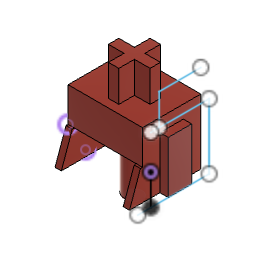
stem v4 (Autodesk Fusion 360 design; units mm, degrees)
Autodesk Fusion 360 part; units mm, degrees
note: some values were not read from the file. Set by a fixed rule: which sketch regions a step uses.
sketch "Sketch1" plane through (0, 0, 0) normal (0, 1, 0) x (1, 0, 0)
  line L0 (0, 0) -> (7.15, 0)
  line L1 (7.15, 0) -> (7.15, -3.3)
  line L2 (7.15, -3.3) -> (0, -3.3)
  line L3 (0, -3.3) -> (0, 0)
  line L4 (0, 0) -> (0.6, 0)
  line L5 (0.6, 0) -> (0.6, 2.95)
  line L6 (0.6, 2.95) -> (0, 2.95)
  line L7 (0, 2.95) -> (0, 0)
  line L8 (7.15, 0) -> (6.55, 0)
  line L9 (6.55, 0) -> (6.55, 2.95)
  line L10 (6.55, 2.95) -> (7.15, 2.95)
  line L11 (7.15, 2.95) -> (7.15, 0)
  dimension "d1" = 7.15
  dimension "d2" = 3.3
  dimension "d3" = 0.6
  dimension "d4" = 2.95
  dimension "d5" = 0.6
  dimension "d6" = 2.95
  constraint horizontal L0
  constraint vertical L1
  constraint horizontal L2
  constraint vertical L3
  constraint coincident L0.start L3.end
  constraint horizontal L4
  constraint vertical L5
  constraint horizontal L6
  constraint vertical L7
  constraint horizontal L8
  constraint vertical L9
  constraint horizontal L10
  constraint vertical L11
  measures "d1" distance of L0.start L0.end
  measures "d2" distance of L0.start L2.end
  measures "d3" distance of L0.start L4.end
  measures "d4" distance of L0.start L6.end
  measures "d5" distance of L0.end L8.end
  measures "d6" distance of L0.end L10.end
extrude "Extrude1" add sketch "Sketch1" along normal blind 5.6
sketch "Sketch2" plane through (7.15, 0, 0) normal (1, 0, 0) x (0, 1, 0)
  line L0 (0, 3.3) -> (0, -2.95)
  line L1 (0, -2.95) -> (5.6, -2.95)
  line L2 (5.6, -2.95) -> (5.6, 3.3)
  line L3 (5.6, 3.3) -> (0, 3.3)
  line L4 (1.675, -2.95) -> (3.925, -2.95)
  line L5 (3.925, -2.95) -> (3.925, 2.05)
  line L6 (3.925, 2.05) -> (1.675, 2.05)
  line L7 (1.675, 2.05) -> (1.675, -2.95)
  point P0 (2.8, 0)
  dimension "d12" = 2.25
  dimension "d13" = 5
  constraint horizontal L4
  constraint vertical L5
  constraint horizontal L6
  constraint vertical L7
  constraint coincident L1 L4.start
  measures "d12" distance of L4.start L4.end
  measures "d13" distance of L4.start L6.end
extrude "Extrude2" add sketch "Sketch2" along normal blind 0.8 contours L1 L4 L5 L6 L7
sketch "Sketch3" plane through (0, 0, 0) normal (-1, 0, 0) x (0, -1, 0)
  line L0 (0, -2.95) -> (0, 3.3)
  line L1 (0, 3.3) -> (-5.6, 3.3)
  line L2 (-5.6, 3.3) -> (-5.6, -2.95)
  line L3 (-5.6, -2.95) -> (0, -2.95)
  line L4 (-1.675, -2.5004) -> (-1.675, -2.95)
  line L5 (-1.675, -2.95) -> (-3.925, -2.95)
  line L6 (-3.925, -2.95) -> (-3.925, -2.5004)
  line L7 (-1.675, -2.95) -> (-3.925, -2.95)
  line L8 (-3.925, -2.95) -> (-3.925, 2.05)
  line L9 (-3.925, 2.05) -> (-1.675, 2.05)
  line L10 (-1.675, 2.05) -> (-1.675, -2.95)
  point P0 (-2.8, -0.0004)
  dimension "d19" = 2.25
  dimension "d20" = 5
  constraint vertical L4
  constraint horizontal L5
  constraint vertical L6
  constraint horizontal L7
  constraint vertical L8
  constraint horizontal L9
  constraint vertical L10
  measures "d19" distance of L6.end L4.start
  measures "d20" distance of L4.end L9.end
extrude "Extrude3" add sketch "Sketch3" along normal blind 0.8 contours L3 L4 L5 L6 L7 L8 L9 L10
sketch "Sketch4" plane through (0, 0, 0) normal (0, -1, 0) x (1, 0, 0)
  line L0 (0.6, -2.95) -> (0.6, 0)
  line L1 (0.6, 0) -> (6.55, 0)
  line L2 (6.55, 0) -> (6.55, -2.95)
  line L3 (6.55, -2.95) -> (7.15, -2.95)
  line L4 (7.15, -2.95) -> (7.15, 3.3)
  line L5 (7.15, 3.3) -> (0, 3.3)
  line L6 (0, 3.3) -> (0, -2.95)
  line L7 (0, -2.95) -> (0.6, -2.95)
  line L8 (0, 0) -> (0.6, 0)
  line L9 (0.6, 0) -> (0.6, -2.95)
  line L10 (0.6, -2.95) -> (0, -2.95)
  line L11 (0, -2.95) -> (0, 0)
  line L12 (6.55, 0) -> (7.15, 0)
  line L13 (7.15, 0) -> (7.15, -2.95)
  line L14 (7.15, -2.95) -> (6.55, -2.95)
  line L15 (6.55, -2.95) -> (6.55, 0)
  constraint horizontal L8
  constraint vertical L9
  constraint horizontal L10
  constraint vertical L11
  constraint coincident L0.start L7.end
  constraint coincident L8.start L11.end
  constraint horizontal L12
  constraint vertical L13
  constraint horizontal L14
  constraint vertical L15
  constraint coincident L3.end L4.start
  constraint coincident L1.end L2.start
extrude "Extrude4" add sketch "Sketch4" along normal blind 2 contours L0 L6 L7 L8 L9 L10 L11 | L2 L3 L4 L12 L13 L14 L15
sketch "Sketch5" plane through (0, 0, 0) normal (-1, 0, 0) x (0, -1, 0)
  line L0 (-3.925, -2.95) -> (-3.925, 2.05)
  line L1 (-3.925, 2.05) -> (-1.675, 2.05)
  line L2 (-1.675, 2.05) -> (-1.675, -2.95)
  line L3 (0, 0) -> (0, 3.3)
  line L4 (0, 3.3) -> (-5.6, 3.3)
  line L5 (-5.6, 3.3) -> (-5.6, -2.95)
  line L6 (-5.6, -2.95) -> (-3.925, -2.95)
sketch "Sketch6" plane through (0, 0, -2.95) normal (0, 0, -1) x (1, 0, 0)
  line L0 (0, 2) -> (0, -1.675)
  line L1 (0, -1.675) -> (-0.8, -1.675)
  line L2 (-0.8, -1.675) -> (-0.8, -3.925)
  line L3 (-0.8, -3.925) -> (0, -3.925)
  line L4 (0, -3.925) -> (0, -5.6)
  line L5 (0, -5.6) -> (0.6, -5.6)
  line L6 (0.6, -5.6) -> (0.6, 2)
  line L7 (0.6, 2) -> (0, 2)
  line L8 (0.6, 2) -> (0, 2)
  line L9 (0, 2) -> (0, 1.4)
  line L10 (0, 1.4) -> (0.6, 1.4)
  line L11 (0.6, 1.4) -> (0.6, 2)
  constraint horizontal L8
  constraint vertical L9
  constraint horizontal L10
  constraint vertical L11
  constraint coincident L0 L9.end
  constraint coincident L6.end L7.start
sketch "Sketch7" plane through (0, 0, -2.95) normal (0, 0, -1) x (1, 0, 0)
  line L0 (6.55, 2) -> (6.55, -5.6)
  line L1 (6.55, -5.6) -> (7.15, -5.6)
  line L2 (7.15, -5.6) -> (7.15, -3.925)
  line L3 (7.15, -3.925) -> (7.95, -3.925)
  line L4 (7.95, -3.925) -> (7.95, -1.675)
  line L5 (7.95, -1.675) -> (7.15, -1.675)
  line L6 (7.15, -1.675) -> (7.15, 2)
  line L7 (7.15, 2) -> (6.55, 2)
  line L8 (7.15, 2) -> (6.55, 2)
  line L9 (6.55, 2) -> (6.55, 1.4)
  line L10 (6.55, 1.4) -> (7.15, 1.4)
  line L11 (7.15, 1.4) -> (7.15, 2)
  dimension "d25" = 0.6
  constraint horizontal L8
  constraint vertical L9
  constraint horizontal L10
  constraint vertical L11
  constraint coincident L6.end L7.start
  measures "d25" distance of L6.end L10.end
extrude "Extrude5" add sketch "Sketch7" sketch "Sketch6" along normal blind 0.5 contours L0 L6 L7 L8 L9 L10 L11 of sketch 2 contours L0 L6 L7 L8 L9 L10 L11
sketch "Sketch8" plane through (0, 0, 0) normal (-1, 0, 0) x (0, -1, 0)
  line L0 (0.2, 0) -> (1.25, -2.95)
  line L1 (1.25, -2.95) -> (1.3, -3.6)
  line L2 (1.3, -3.6) -> (2.5, -3.6)
  line L3 (2.5, -3.6) -> (2.5, 0.457)
  line L4 (2.5, 0.457) -> (0.2, 0)
  constraint horizontal L2
  constraint perpendicular L2 L3
sketch "Sketch9" plane through (0, -1.35, -1.5715) normal (-1, 0, 0) x (0, -1, 0)
extrude "Extrude6" cut sketch "Sketch8" against normal blind 11
sketch "Sketch10" plane through (0, 0, 0) normal (0, 0, -1) x (1, 0, 0)
  line L0 (6.55, 0) -> (0.6, 0)
  line L1 (0.6, 0) -> (0.6, -5.6)
  line L2 (0.6, -5.6) -> (6.55, -5.6)
  line L3 (6.55, -5.6) -> (6.55, 0)
  line L4 (3.575, -5.6) -> (3.575, 0)
  circle A0 centre (3.575, -2.8) radius 1
  circle A1 centre (3.575, -2.8) radius 2
  dimension "d30" = 2
  dimension "d31" = 4
  constraint midpoint L2 L4.start
  constraint midpoint L0 L4.end
  constraint midpoint L4 A0.centre
  constraint concentric A0 A1
  measures "d30" diameter of A0
  measures "d31" diameter of A1
extrude "Extrude7" cut sketch "Sketch10" against normal blind 2 contours L4 A0 A1 | L4 A0 A1
extrude "Extrude8" add 1 faces at (3.8935, 2.8983, 0) along direction (0, 0, -1) blind 5.5
sketch "Sketch11" plane through (0, 0, 0) normal (0, 1, 0) x (1, 0, 0)
fillet "Fillet1" radius 0.25 1 edges at (2.6427, 3.1616, -5.5)
sketch "Sketch12" plane through (0, 0, 3.3) normal (0, 0, 1) x (-1, 0, 0)
  line L0 (0, 0) -> (-7.15, 0)
  line L1 (-7.15, 0) -> (-7.15, -5.6)
  line L2 (-7.15, -5.6) -> (0, -5.6)
  line L3 (0, -5.6) -> (0, 0)
  line L4 (-3.575, -5.6) -> (-3.575, 0)
  line L5 (0, -2.8) -> (-7.15, -2.8)
  line L6 (-1.575, -4.8) -> (-5.575, -4.8)
  line L7 (-5.575, -4.8) -> (-5.575, -0.8)
  line L8 (-5.575, -0.8) -> (-1.575, -0.8)
  line L9 (-1.575, -0.8) -> (-1.575, -4.8)
  line L10 (-1.575, -4.8) -> (-5.575, -0.8) construction
  line L11 (-5.575, -4.8) -> (-1.575, -0.8) construction
  line L12 (-3.075, -4.8) -> (-4.075, -4.8)
  line L13 (-4.075, -4.8) -> (-4.075, -0.8)
  line L14 (-4.075, -0.8) -> (-3.075, -0.8)
  line L15 (-3.075, -0.8) -> (-3.075, -4.8)
  line L16 (-3.075, -4.8) -> (-4.075, -0.8) construction
  line L17 (-4.075, -4.8) -> (-3.075, -0.8) construction
  line L18 (-1.575, -3.3) -> (-5.575, -3.3)
  line L19 (-5.575, -3.3) -> (-5.575, -2.3)
  line L20 (-5.575, -2.3) -> (-1.575, -2.3)
  line L21 (-1.575, -2.3) -> (-1.575, -3.3)
  line L22 (-1.575, -3.3) -> (-5.575, -2.3) construction
  line L23 (-5.575, -3.3) -> (-1.575, -2.3) construction
  point P0 (-3.575, -2.8)
  point P1 (-3.575, -2.8)
  point P2 (-3.575, -2.8)
  dimension "d38" = 4
  dimension "d39" = 4
  dimension "d40" = 1
  dimension "d41" = 4
  dimension "d42" = 4
  dimension "d43" = 1
  constraint midpoint L2 L4.start
  constraint midpoint L0 L4.end
  constraint midpoint L3 L5.start
  constraint midpoint L1 L5.end
  constraint horizontal L6
  constraint perpendicular L6 L7
  constraint parallel L6 L8
  constraint parallel L7 L9
  constraint coincident L10 P2
  constraint coincident L11 P2
  constraint midpoint L4 P2
  constraint horizontal L12
  constraint perpendicular L12 L13
  constraint parallel L12 L14
  constraint parallel L13 L15
  constraint coincident L16 P2
  constraint coincident L17 P2
  constraint coincident P2 P1
  constraint horizontal L18
  constraint perpendicular L18 L19
  constraint parallel L18 L20
  constraint parallel L19 L21
  constraint coincident L22 P2
  constraint coincident L23 P2
  measures "d38" distance of L7.end L8.end
  measures "d39" distance of L6.end L7.end
  measures "d40" distance of L13.end L14.end
  measures "d41" distance of L12.end L13.end
  measures "d42" distance of L19.end L20.end
  measures "d43" distance of L18.end L19.end
extrude "Extrude9" add sketch "Sketch12" along normal blind 3 contours L4 L8 L14 L15 L20 | L4 L8 L13 L14 L20 | L5 L9 L15 L18 L21 | L5 L9 L15 L20 L21 | L4 L5 L15 L20 | L4 L5 L13 L20 | L4 L5 L15 L18 | L5 L7 L13 L19 L20 | L5 L7 L13 L18 L19 | L4 L5 L13 L18 | L4 L6 L12 L13 L18 | L4 L6 L12 L15 L18
sketch "Sketch13" plane through (0, 0, 0) normal (1, 0, 0) x (0, 1, 0)
sketch "Sketch14" plane through (0, 0, -5.5) normal (0, 0, -1) x (1, 0, 0)
  circle A0 centre (3.575, -2.8) radius 0.75
sketch "Sketch15" plane through (7.95, 0, 0) normal (1, 0, 0) x (0, 1, 0)
  line L0 (1.675, 2.05) -> (1.675, -2.95)
  line L1 (1.675, -2.95) -> (3.925, -2.95)
  line L2 (3.925, -2.95) -> (3.925, 2.05)
  line L3 (3.925, 2.05) -> (1.675, 2.05)
  line L4 (0.8, 6.3) -> (4.8, 6.3)
  line L5 (0.8, 6.3) -> (0.8, 3.3)
  line L6 (0, 3.3) -> (5.6, 3.3)
  line L7 (5.6, 3.3) -> (5.6, -2.95)
  line L8 (5.6, -2.95) -> (5.6, 3.3)
  line L9 (-1.25, -2.95) -> (5.6, -2.95)
  line L10 (0, 0) -> (0, -2.95)
  dimension "d46" = 4
  dimension "d47" = 3
  dimension "d48" = 5.6
  dimension "d49" = 6.25
  dimension "d50" = 6.85
  dimension "d51" = 2.95
  constraint horizontal L4
  constraint perpendicular L4 L5
  constraint horizontal L6
  constraint perpendicular L6 L7
  constraint perpendicular L6 L8
  constraint perpendicular L7 L9
  constraint coincident L10.start origin
  constraint perpendicular L9 L10
  measures "d46" distance of L4.start L4.end
  measures "d47" distance of L4.start L5.end
  measures "d48" distance of L6.start L6.end
  measures "d49" distance of L7.end L6.end
  measures "d50" distance of L9.start L7.end
  measures "d51" distance of L10.start L10.end
